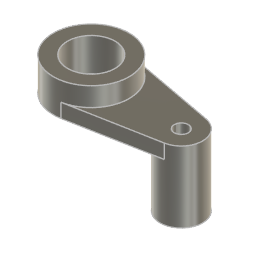
Practice problem 3 (Solid works) (Autodesk Fusion 360 design; units mm, degrees)
Autodesk Fusion 360 part; units mm, degrees
sketch "Sketch1" plane through (0, 0, 0) normal (0, 0, 1) x (1, 0, 0)
  circle A0 centre (0, 0) radius 10
  line L0 (0, 10) -> (0, -10) construction
  line L1 (0, 0) -> (38, 0) construction
  circle A1 centre (38, 0) radius 3
  circle A2 centre (38, 0) radius 9
  circle A3 centre (0, 0) radius 16
  line L2 (2.9474, 15.7262) -> (39.6579, 8.846)
  line L3 (2.9474, -15.7262) -> (39.6579, -8.846)
  dimension "d1" = 20
  dimension "d2" = 38
  dimension "d3" = 6
  dimension "d4" = 18
  dimension "d5" = 32
  constraint coincident A0.centre L1.start
  constraint coincident A0 L0.start
  constraint coincident A0 L0.end
  constraint vertical L0
  constraint perpendicular L0 L1
  constraint coincident L1.end A1.centre
  constraint concentric A1 A2
  constraint coincident A3 L2.start
  constraint coincident A2 L2.end
  constraint tangent A2 L2
  constraint tangent A3 L2
  constraint coincident A3 L3.start
  constraint coincident A2 L3.end
  constraint tangent A2 L3
  constraint tangent A3 L3
  measures "d1" diameter of A0
  measures "d2" distance of A0.centre L1.end
  measures "d3" diameter of A1
  measures "d4" diameter of A2
  measures "d5" diameter of A3
extrude "Extrude1" add sketch "Sketch1" along normal blind 14 contours A3
extrude "Extrude2" add sketch "Sketch1" along normal blind 6 contours A2 A3 L2 L3
extrude "Extrude3" add sketch "Sketch1" along normal blind 6 contours A2
extrude "Extrude4" add sketch "Sketch1" against normal blind 24 contours A2
